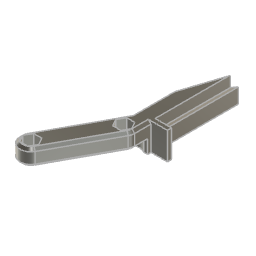
_ConnectorArmV2_left.0cba4ef7-d469-4558-aa08-ed3d96de5736 (Autodesk Fusion 360 design; units mm, degrees)
Autodesk Fusion 360 part; units mm, degrees
other "Derived from MasterParameters_Gripper v74"
sketch "Sketch1" plane through (0, 0, 0) normal (0, 0, 1) x (1, 0, 0)
  circle A0 centre (0, 0) radius 3.95
  circle A1 centre (-12, -22) radius 3.95
  circle A2 centre (-12, -22) radius 1.45
  circle A3 centre (0, 0) radius 1.45
  line L0 (3.4677, -1.8915) -> (-8.5323, -23.8915)
  line L1 (-3.5352, 1.7676) -> (-15.4677, -20.1085)
  line L2 (3.95, 0) -> (3.95, 35)
  line L3 (3.95, 35) -> (0.95, 35)
  line L4 (0.95, 35) -> (-3.95, 20)
  line L5 (-3.95, 0) -> (-3.95, 20)
  line L6 (1.4722, -2.55) -> (2.9445, 0)
  line L7 (2.9445, 0) -> (1.4722, 2.55)
  line L8 (1.4722, 2.55) -> (-1.4722, 2.55)
  line L9 (-1.4722, 2.55) -> (-2.9445, 0)
  line L10 (-2.9445, 0) -> (-1.4722, -2.55)
  line L11 (-1.4722, -2.55) -> (1.4722, -2.55)
  line L12 (-10.5278, -24.55) -> (-9.0555, -22)
  line L13 (-9.0555, -22) -> (-10.5278, -19.45)
  line L14 (-10.5278, -19.45) -> (-13.4722, -19.45)
  line L15 (-13.4722, -19.45) -> (-14.9445, -22)
  line L16 (-14.9445, -22) -> (-13.4722, -24.55)
  line L17 (-13.4722, -24.55) -> (-10.5278, -24.55)
  point P0 (-12, -22)
  constraint coincident A0.centre A3.centre
  constraint concentric A1 A2
  constraint equal A2 A3
  constraint equal A0 A1
  constraint coincident A0 L0.start
  constraint coincident A1 L0.end
  constraint tangent A1 L0
  constraint coincident A1 L1.end
  constraint tangent A1 L1
  constraint tangent A0 L0
  constraint perpendicular L2 L3
  constraint tangent A0 L2
  constraint tangent A0 L1
  constraint vertical L5
  constraint tangent A0 L5
  constraint coincident A0 L5.start
  constraint parallel L2 L5
  constraint coincident A0 L2.start
  constraint coincident P0 A1.centre
  constraint horizontal L17
  constraint equal L11 L17
  constraint horizontal L11
  measures "d1" distance of A0.centre A1.centre
  measures "d30" diameter of A3
  measures "d31" distance of A1 A2
  measures "d32" distance of P0 A0.centre
  measures "d54" distance of L5.start L4.end
  measures "d59" distance of L3.end L4.end
  measures "d61" distance of L2.end L3.end
  measures "d73" distance of L14 L17
extrude "Extrude1" add sketch "Sketch1" along normal blind 6 contours A0 | A0 L2 L3 L4 L5 | A0 A1 L0 L1 L5 | A1 | L6 L7 L8 L9 L10 L11 | L12 L13 L14 L15 L16 L17
sketch "Sketch6" plane through (0, 0, 0) normal (0, 0, -1) x (1, 0, 0)
  circle A0 centre (-12, 22) radius 1.45
  circle A1 centre (0, 0) radius 1.45
  line L0 (3.95, -35) -> (3.95, 0)
  arc A2 (3.95, 0) -> (3.4677, 1.8915) centre (0, 0) ccw
  line L1 (3.4677, 1.8915) -> (-8.5323, 23.8915)
  arc A3 (-8.5323, 23.8915) -> (-15.4677, 20.1085) centre (-12, 22) ccw
  line L2 (-15.4677, 20.1085) -> (-3.95, -1.0072)
  line L3 (-3.95, -1.0072) -> (-3.95, -20)
  line L4 (-3.95, -20) -> (0.95, -35)
  line L5 (0.95, -35) -> (3.95, -35)
  arc A4 (-2.6105, -4.7271) -> (2.6105, -4.7271) centre (0, 0) ccw
  line L6 (0, 0) -> (0, -5.4) construction
  line L7 (2.6105, -4.7271) -> (3.95, -4.7271)
  line L8 (-2.6105, -4.7271) -> (-3.95, -4.7271)
  line L9 (-3.95, -1.0072) -> (-3.95, -20)
  line L10 (3.95, 0) -> (3.95, -35)
  line L11 (3.95, -35) -> (0.95, -35)
  line L12 (0.95, -35) -> (-3.95, -20)
  dimension "d70" = 5.4
  constraint coincident A1.centre A2.centre
  constraint midpoint A4 L6.end
  constraint vertical L6
  constraint coincident L0 L7.end
  constraint perpendicular L0 L7
  constraint coincident L3 L8.end
  constraint perpendicular L3 L8
  measures "d70" distance of A1.centre L6.end
extrude "Extrude6" add sketch "Sketch6" along normal blind 4 contours L0 L3 L4 L5 A4 L7 L8 L9 L10 L11 L12
sketch "Sketch3" plane through (0, 35, 0) normal (0, 1, 0) x (-1, 0, 0)
  line L0 (-0.95, -4) -> (-0.95, 6)
  line L1 (-0.95, 6) -> (-3.95, 6)
  line L2 (-3.95, 6) -> (-3.95, -4)
  line L3 (-3.95, 1) -> (-6.8921, 1) construction
  line L4 (-6.8921, -1.7211) -> (-6.8921, 3.7211)
  line L5 (-6.8921, 3.7211) -> (-3.95, 2.041)
  line L6 (-6.8921, -1.7211) -> (-3.95, -0.041)
  line L7 (-3.95, -4) -> (-0.95, -4)
  constraint midpoint L2 L3.start
  constraint perpendicular L2 L3
  constraint perpendicular L3 L4
  constraint coincident L3.end L4
  constraint midpoint L3.end L4
  constraint coincident L2 L5.end
  constraint symmetric L3 L4.end L4.start
  constraint symmetric L3 L5.end L6.end
sketch "Sketch4" plane through (3.95, 0, 0) normal (1, 0, 0) x (0, 1, 0)
  line L0 (35, -4) -> (35, 6)
  line L1 (35, 6) -> (0, 6)
  line L2 (0, 6) -> (0, 0)
  line L3 (0, 0) -> (4.7271, 0)
  line L4 (6, 6) -> (7.5, 6)
  line L5 (7.5, 6) -> (7.5, -4)
  line L6 (6, -4) -> (6, 6)
  line L7 (0, 6) -> (35, 6)
  line L8 (0, 0) -> (4.7271, 0)
  line L9 (4.7271, 0) -> (4.7271, -4)
  line L10 (4.7271, -4) -> (35, -4)
  dimension "d48" = 1.5
  dimension "d55" = 6
  constraint horizontal L4
  constraint vertical L5
  constraint vertical L6
  constraint coincident L4.start L6.end
  constraint coincident L1 L4.start
  constraint coincident L6.start L10
  constraint coincident L5.end L10
  measures "d48" distance of L5 L6
  measures "d55" distance of L2 L6
extrude "Extrude3" add sketch "Sketch4" along normal blind 6 contours L1 L4 L5 L6 L7 L10
extrude "Extrude4" add sketch "Sketch3" against normal up to surface (27.5 mm away) contours L2 L4 L5 L6
extrude "Extrude5" cut sketch "Sketch1" against normal blind 3.8 from surface at 6 contours L6 L7 L8 L9 L10 L11 | L12 L13 L14 L15 L16 L17
chamfer "Chamfer1" distance 3 angle 45 4 edges at (-3.95, 10.5036, 6) (-1.5, 27.5, 6) (-3.95, 12.3635, -4) (-1.5, 27.5, -4)
chamfer "Chamfer2" distance 1 angle 45 10 edges at (-8.2088, -6.8007, 6) (-13.8915, -25.4677, 6) (-2.5323, -12.8915, 6) (3.8275, -0.976, 6) (3.95, 3, 6) (-9.7088, -9.5507, 0) (-13.8915, -25.4677, 0) (-2.5323, -12.8915, 0) (3.8275, -0.976, 0) (3.95, 2.3635, 0)
equation "d1 = plate_distance_back_front_y_Ref"
equation "m2_nut_diameter_Ref = 4.2 mm"
equation "m2_nut_height_Ref = 3 mm"
equation "arm_screw_wall_thickness_Ref = 1 mm"
equation "m2_screw_diameter_Ref = 2.2 mm" comment "diameter with tolerance"
equation "m25_screw_diameter_Ref = 2.7 mm"
equation "m25_wall_thickness_Ref = 2 mm"
equation "m2_tapping_tolerance_Ref = 0.2 mm"
equation "Servo_cut_gap_Ref = 0.5 mm"
equation "m25_screw_head_height_Ref = 2.5 mm"
equation "m25_screw_head_width_Ref = 4.6 mm"
equation "m25_arm_screw_plus_tolerance_Ref = 2.9 mm" comment "Additional parameter to experiment with parameter to hopefully enable free movement of arm"
equation "m2_tapping_head_width_Ref = 4.4 mm"
equation "back_arms_thickness_Ref = 8.5 mm"
equation "m2_screw_head_diameter_Ref = 4 mm"
equation "m2_screw_head_height_Ref = 2 mm"
equation "arm_height_Ref = 4 mm"
equation "arm_ground_clearance_Ref = 1 mm"
equation "m3_screw_diameter_Ref = 3.2 mm"
equation "m3_wall_thickness_gripper_mount_Ref = 2 mm"
equation "arm_length_Ref = 35 mm"
equation "gear_arm_gap_Ref = 0.05 mm"
equation "distance_lower_upper_plate_Ref = 10 mm"
equation "gear_screw_dist_Ref = 1.5 mm"
equation "gear_z_height_placement_on_arm_Ref = 5 mm"
equation "plate_distance_back_axes_Ref = 30 mm" comment "Distance between back-axes, namely servo and the arm axis of the arm in the back"
equation "distance_arms_front_Ref = 12 mm" comment "Distance from the back to the front axis"
equation "d30 = m25_arm_screw_plus_tolerance_Ref"
equation "d31 = m25_wall_thickness_Ref + 0.5 mm"
equation "d32 = distance_arms_front_Ref"
equation "d33 = arm_height_Ref + 2 mm"
equation "gear_arm_connector_height_Ref = 4 mm"
equation "m25_ruthex_outer_Ref = 7.2 mm"
equation "m25_ruthex_inner_Ref = 4 mm"
equation "m25_ruthex_height_Ref = 5.7 mm"
equation "plate_single_height_Ref = 3 mm" comment "height of a single plate piece"
equation "plate_distance_back_front_y_Ref = 22 mm"
equation "stand_width_Ref = 5 mm" comment "width of the stand that the gripper can be mounted onto"
equation "gripper_tpu_thickness_Ref = 6 mm"
equation "d53 = gripper_tpu_thickness_Ref"
equation "arm_top_tolerance_Ref = 0.2 mm"
equation "gear_square_length_Ref = 5.9 mm"
equation "m25_nyloc_width_Ref = 5.1 mm"
equation "m25_nyloc_height_Ref = 3.8 mm"
equation "d66 = -m25_nyloc_height_Ref"
equation "d70 = m25_arm_screw_plus_tolerance_Ref + m25_wall_thickness_Ref + 0.5 mm"
equation "d73 = m25_nyloc_width_Ref"
